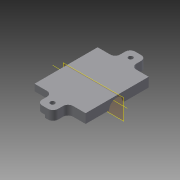
# Autodesk Inventor part: bnc-mount
Saved by Autodesk Inventor 2015 SP1 (Build 190203100, 203)
## iProperties
Created: 2015-04-03
Part Number: bnc-mount
Material: Generic
Document SubType Name: Modeling
Designer: kam42
Density: 1 g/cm^3
Appearance: Default
Author: kam42
Autodesk Inventor part; units mm, degrees
ref_plane "YZ Plane" through (0, 0, 0) normal (1, 0, 0) x (0, 1, 0)
ref_plane "XZ Plane" through (0, 0, 0) normal (0, 1, 0) x (-1, 0, 0)
ref_plane "XY Plane" through (0, 0, 0) normal (0, 0, 1) x (1, 0, 0)
sketch "Sketch1" plane through (0, 0, 0) normal (0, 0, 1) x (1, 0, 0)
  line L0 (0, 0) -> (0, 59.9999)
  line L1 (0, 59.9999) -> (45.0012, 59.9999)
  line L2 (45.0012, 59.9999) -> (45.0012, 0)
  line L3 (45.0012, 0) -> (0, 0)
  circle A0 centre (29.9999, 52.4993) radius 3.175
  circle A1 centre (29.9999, 7.5006) radius 3.175
  circle A2 centre (5.4991, 54.5008) radius 0.5842
  circle A3 centre (2.1996, 57.8002) radius 1.0541
  circle A4 centre (8.8011, 57.8002) radius 1.0541
  circle A5 centre (8.8011, 51.1988) radius 1.0541
  circle A6 centre (2.1996, 51.1988) radius 1.0541
  circle A7 centre (5.4991, 29.9999) radius 0.5842
  circle A8 centre (2.1996, 33.2994) radius 1.0541
  circle A9 centre (8.8011, 33.2994) radius 1.0541
  circle A10 centre (2.1996, 26.7005) radius 1.0541
  circle A11 centre (5.4991, 5.4991) radius 0.5842
  circle A12 centre (2.1996, 8.8011) radius 1.0541
  circle A13 centre (8.8011, 8.8011) radius 1.0541
  circle A14 centre (8.8011, 2.1996) radius 1.0541
  circle A15 centre (2.1996, 2.1996) radius 1.0541
  circle A16 centre (41.0312, 34.4602) radius 0.4496
  circle A17 centre (41.0312, 31.9202) radius 0.4496
  circle A18 centre (41.0312, 29.3802) radius 0.4496
  circle A19 centre (41.0312, 26.8402) radius 0.4496
  circle A20 centre (41.0312, 24.3002) radius 0.4496
  circle A21 centre (30.0939, 24.9352) radius 0.4496
  circle A22 centre (32.6339, 24.9352) radius 0.4496
  circle A23 centre (8.8011, 26.7005) radius 1.0541
  line L4 (45.5012, 60.4999) -> (45.5012, -0.5)
  line L5 (45.5012, -0.5) -> (-0.5, -0.5)
  line L6 (-0.5, -0.5) -> (-0.5, 60.4999)
  line L7 (-0.5, 60.4999) -> (45.5012, 60.4999)
  dimension "d0" = 0.5
  constraints: 24 centre point, 16 end point, 2 horizontal, 2 vertical, 1 coincident, 56 other
  measures "d0" distance between parallel lines of L7 L1
extrude "Extrusion1" add sketch "Sketch1" against normal blind 1 contours L0 L1 L2 L3 | A0 | A1 | A2 | A3 | A4 | A5 | A6 | A7 | A8 | A9 | A10 | A11 | A12 | A13 | A14 | A15 | A16 | A17 | A18 | A19 | A20 | A21 | A22 | A23 | L4 L5 L6 L7
sketch "Sketch2" plane through (0, 0, 0) normal (0, 0, 1) x (1, 0, 0)
  circle A0 centre (29.9999, 52.4993) radius 3.175 projected
  circle A1 centre (29.9999, 7.5006) radius 3.175 projected
  circle A2 centre (29.9999, 52.4993) radius 2.675
  circle A3 centre (29.9999, 7.5006) radius 2.675
  point P0 (0, 0)
  dimension "d6" = 0.5
  dimension "d8" = 0.5
  constraints: 2 centre point
  measures "d6" radial gap between concentric circles of A0 A2
  measures "d8" radial gap between concentric circles of A1 A3
extrude "Extrusion2" add sketch "Sketch2" along normal blind 8.25 contours A2 | A3
sketch "Sketch3" plane through (0, 0, 0) normal (0, 0, 1) x (1, 0, 0)
  line L0 (45.5012, 60.4999) -> (45.5012, -0.5) projected
  line L1 (-0.5, 60.4999) -> (45.5012, 60.4999) projected
  line L2 (-0.5, -0.5) -> (-0.5, 60.4999) projected
  line L3 (45.5012, -0.5) -> (-0.5, -0.5) projected
  line L4 (46.5012, 61.4999) -> (46.5012, -1.5)
  line L5 (46.5012, -1.5) -> (-1.5, -1.5)
  line L6 (-1.5, -1.5) -> (-1.5, 61.4999)
  line L7 (-1.5, 61.4999) -> (46.5012, 61.4999)
  line L8 (-1.5, 61.4999) -> (-4.5, 61.4999)
  line L9 (-4.5, 61.4999) -> (-4.5, -1.5)
  line L10 (-4.5, -1.5) -> (-1.5, -1.5)
  line L11 (-1.5, -1.5) -> (-1.5, 61.4999)
  point P0 (0, 0)
  dimension "d11" = 1
  dimension "d40" = 3
  constraints: 16 end point, 2 parallel, 1 horizontal, 1 perpendicular, 3 other
  measures "d11" distance between parallel lines of L1 L7
  measures "d40" distance of L9.end L10.end
extrude "Extrusion3" add sketch "Sketch3" along normal blind 16.5 and the other way blind 1
sketch "Sketch5" plane through (-4.5, -1.5, 16.5) normal (-1, 0, 0) x (0, 0, 1)
  line L0 (-16.5, 56.6743) -> (-16.5, 51.3243)
  line L1 (-16.5, 11.6756) -> (-16.5, 6.3256)
  line L2 (-16.5, 61.9999) -> (-16.5, 1)
  line L3 (-16.5, 1) -> (-16.5, 61.9999)
  circle A0 centre (-5.5, 56.0008) radius 5
  circle A1 centre (-5.5, 31.4999) radius 5
  circle A2 centre (-5.5, 6.9991) radius 5
  line L4 (-10.5, 56.0008) -> (-10.5, 6.9991) construction
  point P0 (-16.5, 1.5)
  point P1 (-16.5, 31.4999)
  point P2 (-16.5, 56.0008)
  point P3 (-16.5, 6.9991)
  point P4 (-16.5, 31.4999)
  dimension "d16" = 10
  dimension "d18" = 10
  dimension "d17" = 10
  dimension "d20" = 6
  constraints: 10 end point, 5 horizontal alignment, 2 vertical, 2 vertical alignment, 1 centre point, 1 midpoint, 4 other
  measures "d17" diameter of A1
  measures "d20" distance between parallel lines of L2 L4
sketch "Sketch6" plane through (0, 0, 0) normal (0, 0, 1) x (1, 0, 0)
  line L0 (-0.5, -0.5) -> (-0.5, 60.4999) projected
  line L1 (-0.5, 48.2508) -> (11.5, 48.2508)
  line L2 (11.5, 48.2508) -> (11.5, 36.2508)
  line L3 (11.5, 36.2508) -> (-0.5, 36.2508)
  line L4 (-0.5, 36.2508) -> (-0.5, 48.2508)
  line L5 (-0.5, 23.7499) -> (11.5, 23.7499)
  line L6 (11.5, 23.7499) -> (11.5, 11.7499)
  line L7 (11.5, 11.7499) -> (-0.5, 11.7499)
  line L8 (-0.5, 11.7499) -> (-0.5, 23.7499)
  line L9 (-0.5, 48.2508) -> (11.5, 36.2508) construction
  line L10 (-0.5, 36.2508) -> (11.5, 48.2508) construction
  line L11 (-0.5, 23.7499) -> (11.5, 11.7499) construction
  line L12 (11.5, 23.7499) -> (-0.5, 11.7499) construction
  point P0 (0, 0)
  point P1 (5.5, 42.2508)
  point P2 (5.5, 17.7499)
  point P3 (5.4991, 29.9999)
  point P4 (5.4991, 54.5008)
  dimension "d21" = 12
  dimension "d22" = 12
  dimension "d23" = 12
  dimension "d24" = 12.25
  dimension "d25" = 12.25
  constraints: 24 end point, 4 parallel, 4 point on line, 3 perpendicular, 2 horizontal, 2 midpoint
  measures "d21" distance of L5.end L6.end
  measures "d22" distance of L1.end L2.end
  measures "d23" distance of L5.start L5.end
  measures "d24" distance of point (5.499, 30) point (5.5, 17.75)
  measures "d25" distance of point (5.499, 54.501) point (5.5, 42.251)
extrude "Extrusion4" add sketch "Sketch6" along normal blind 3.75
extrude "Extrusion5" cut sketch "Sketch5" against normal up to surface (4 mm away)
sketch "Sketch7" plane through (46.5012, -1.5, 16.5) normal (1, 0, 0) x (0, 0, -1)
  line L0 (16.5, 61.9999) -> (16.5, 1) projected
  circle A0 centre (8.5, 30.8802) radius 2
  point P0 (16.5, 1.5)
  point P1 (16.5, 30.8802)
  point P2 (10.5, 30.8802)
  dimension "d33" = 4
  dimension "d32" = 6
  constraints: 1 horizontal alignment, 2 other
  measures "d32" distance of point (10.5, 30.88) point (16.5, 30.88)
extrude "Extrusion6" cut sketch "Sketch7" against normal up to surface (1 mm away)
sketch "Sketch8" plane through (0, 0, 16.5) normal (0, 0, 1) x (1, 0, 0)
  line L0 (45.5012, -0.5) -> (-0.5, -0.5) projected
  line L1 (-0.5, -0.5) -> (-0.5, 60.4999) projected
  line L2 (-0.5, 60.4999) -> (45.5012, 60.4999) projected
  line L3 (45.5012, 60.4999) -> (45.5012, -0.5) projected
  line L4 (46.5012, 61.4999) -> (-4.5, 61.4999) projected
  line L5 (-4.5, 61.4999) -> (-4.5, -1.5) projected
  line L6 (-4.5, -1.5) -> (46.5012, -1.5) projected
  line L7 (46.5012, -1.5) -> (46.5012, 61.4999) projected
  point P0 (0, 0)
extrude "Extrusion8" add sketch "Sketch8" along normal blind 1 contours L0 L1 L2 L3 | L7 L6 L5 L4
ref_plane "Work Plane1" through (-3.5, -1.5, 16.5) normal (0, -1, 0) x (1, 0, 0)
sketch "Sketch10" plane through (-3.5, -1.5, 16.5) normal (0, -1, 0) x (1, 0, 0)
  line L0 (24.5006, -5.5) -> (24.5006, -8.25)
  line L1 (50.0012, -8.25) -> (24.5006, -8.25)
  line L2 (-1, -5.5) -> (24.5006, -5.5)
  line L3 (50.0012, -6.5) -> (50.0012, -10.5) projected
  line L4 (-1, -10.5) -> (-1, -0.5) projected
  line L5 (3, -0.5) -> (3, -10.5) projected
  constraints: 6 end point, 1 horizontal, 1 parallel
split body "Split1" sketch "Sketch10" result two bodies curves L1 L0 L2 first body at (12.5004, 40.4999, -0.5)
ref_plane "Work Plane2" through (46.5012, -0.5, 0) normal (1, 0, 0) x (0, 0, -1)
sketch "Sketch13" plane through (46.5012, -0.5, 0) normal (1, 0, 0) x (0, 0, -1)
  line L0 (-8.25, -1) -> (-8.25, 27.8959) projected
  line L1 (-8.25, -1) -> (1, -1) projected
  line L2 (1, 61.9999) -> (1, -1) projected
  line L3 (1, 61.9999) -> (-8.25, 61.9999) projected
  line L4 (-8.25, 31.8645) -> (-8.25, 61.9999) projected
  arc A0 (-6, 29.8802) -> (-8.25, 31.8645) centre (-8, 29.8802) ccw projected
  arc A1 (-8.25, 27.8959) -> (-6, 29.8802) centre (-8, 29.8802) ccw projected
  circle A2 centre (-8, 29.8802) radius 5
  circle A3 centre (-8, 29.8802) radius 2
  line L5 (-8.25, 27.8959) -> (-8.25, 0) projected
  line L6 (-8.25, 24.8864) -> (-8.25, 27.8959)
  line L7 (-8.25, 31.8645) -> (-8.25, 34.8739)
  line L8 (-8.25, 31.8645) -> (-8.25, 61.9999) projected
  dimension "d63" = 10
  constraints: 4 end point, 2 centre point, 2 coincident, 2 point on circle, 2 point on line, 1 collinear
  measures "d63" diameter of A2
extrude "Extrusion14" add sketch "Sketch13" along normal blind 4 contours L0 A1 A0 L4 A2 bodies 2
sketch "Sketch18" plane through (46.5012, -1.5, 17.5) normal (1, 0, 0) x (0, 0, -1)
  line L0 (9.25, 0) -> (9.25, 28.8959) projected
  arc A0 (9.25, 32.8645) -> (9.25, 28.8959) centre (9.5, 30.8802) ccw projected
  line L1 (9.25, 32.8645) -> (9.25, 62.9999) projected
  arc A1 (9.25, 25.8864) -> (9.25, 35.8739) centre (9.5, 30.8802) ccw projected
  circle A2 centre (9.5, 30.8802) radius 7.5
  circle A3 centre (9.5, 30.8802) radius 2
  line L2 (9.25, 25.8864) -> (9.25, 28.8959)
  line L3 (9.25, 28.8959) -> (9.25, 1) projected
  line L4 (9.25, 35.8739) -> (9.25, 32.8645)
  point P0 (17.5, 1.5)
  dimension "d140" = 15
  constraints: 4 end point, 2 centre point, 2 coincident, 2 collinear
  measures "d140" diameter of A2
sketch "Sketch21" plane through (-4.5, -1.5, -1) normal (0, -1, 0) x (1, 0, 0)
  line L0 (25.5006, 9.25) -> (51.0012, 9.25) projected
  line L1 (25.5006, 12) -> (25.5006, 9.25) projected
  line L2 (51.0012, 0) -> (0, 0) projected
  line L3 (4, 12) -> (25.5006, 12) projected
  line L4 (17.5006, 12) -> (25.5006, 12)
  line L5 (33.5006, 9.25) -> (33.5006, 0)
  line L6 (33.5006, 0) -> (17.5006, 0)
  line L7 (17.5006, 0) -> (17.5006, 12)
  point P0 (4.5, 1)
  dimension "d78" = 8
  dimension "d79" = 8
  constraints: 8 end point, 4 point on line, 2 parallel, 1 horizontal, 1 perpendicular
  measures "d78" distance between parallel lines of L1 L7
  measures "d79" distance between parallel lines of L5 L1
extrude "Extrusion18" add sketch "Sketch21" along normal blind 15 bodies 2
sketch "Sketch22" plane through (-4.5, -1.5, 17.5) normal (0, -1, 0) x (1, 0, 0)
  line L0 (25.5006, -6.5) -> (25.5006, -9.25) projected
  line L1 (25.5006, -9.25) -> (25.5006, -6.5) projected
  line L2 (25.5006, -6.5) -> (17.5006, -6.5) projected
  line L3 (17.5006, -6.5) -> (17.5006, -18.5) projected
  line L4 (17.5006, -18.5) -> (33.5006, -18.5) projected
  line L5 (33.5006, -18.5) -> (33.5006, -9.25) projected
  line L6 (33.5006, -9.25) -> (25.5006, -9.25) projected
  line L7 (51.0012, 0) -> (0, 0) projected
  line L8 (33.5006, -9.25) -> (25.5006, -9.25)
  line L9 (17.5006, -6.5) -> (17.5006, 0)
  line L10 (17.5006, 0) -> (33.5006, 0)
  line L11 (33.5006, 0) -> (33.5006, -9.25)
  line L12 (17.5006, -6.5) -> (25.5006, -6.5)
  point P0 (4.5, -17.5)
  constraints: 10 end point, 3 point on line, 2 horizontal, 2 parallel, 1 perpendicular
extrude "Extrusion19" add sketch "Sketch22" along normal blind 15 contours L2 L9 L7 L11 L6 L0 bodies 3
sketch "Sketch23" plane through (0, 0, 17.5) normal (0, 0, 1) x (1, 0, 0)
  line L0 (21.0006, -0.5) -> (21.0006, -16.5) projected
  point P0 (0, 0)
  point P1 (21.0006, -9)
  constraints: 1 point on line
hole "Hole1" at (21.0006, -9, 17.5) direction (0, 0, -1) diameter 4.4958 end through all bodies 3 2
sketch "Sketch24" plane through (0, 0, -1) normal (0, 0, -1) x (-1, 0, 0)
  circle A0 centre (-21.0006, -9) radius 2.2479 projected
  line L0 (-25.3381, -11.5367) -> (-25.3662, -6.5119)
  line L1 (-25.3662, -6.5119) -> (-21.0287, -3.9752)
  line L2 (-21.0287, -3.9752) -> (-16.663, -6.4633)
  line L3 (-16.663, -6.4633) -> (-16.635, -11.4881)
  line L4 (-16.635, -11.4881) -> (-20.9725, -14.0248)
  line L5 (-20.9725, -14.0248) -> (-25.3381, -11.5367)
  point P0 (0, 0)
  dimension "d91" = 8.7312
  constraints: 12 end point, 1 coincident, 13 other
  measures "d91" horizontal distance of L0.end L3.end
extrude "Extrusion20" cut sketch "Sketch24" against normal blind 3.175 bodies 2
ref_plane "Work Plane4" through (-4.5, 29.9999, 11) normal (0, -1, 0) x (1, 0, 0)
mirror "Mirror2" about plane through (-4.5, 29.9999, 11) normal (0, -1, 0) of "Extrusion18", "Hole1", "Extrusion20" bodies 2
mirror "Mirror3" about plane through (-4.5, 29.9999, 11) normal (0, -1, 0) of "Extrusion19", "Hole1" bodies 3
fillet "Fillet4" radius 5 16 edges at (13.0006, -1.5, 5) (13.0006, -16.5, 5) (29.0006, -16.5, 3.625) (29.0006, -1.5, 3.625) (13.0006, 61.4999, 5) (13.0006, 76.4999, 5) (29.0006, 76.4999, 3.625) (29.0006, 61.4999, 3.625) (13.0006, -1.5, 14.25) (13.0006, -16.5, 14.25) (29.0006, -16.5, 12.875) (29.0006, -1.5, 12.875) (13.0006, 61.4999, 14.25) (13.0006, 76.4999, 14.25) (29.0006, 76.4999, 12.875) (29.0006, 61.4999, 12.875)
sketch "Sketch25" plane through (0, 0, 0) normal (0, 0, 1) x (1, 0, 0)
  circle A0 centre (29.9999, 7.5006) radius 2.675 projected
  circle A1 centre (29.9999, 52.4993) radius 2.675 projected
  circle A2 centre (29.9999, 52.4993) radius 5
  circle A3 centre (29.9999, 7.5006) radius 5
  point P0 (0, 0)
  dimension "d96" = 10
  dimension "d97" = 10
  constraints: 2 centre point, 2 coincident
  measures "d96" diameter of A2
  measures "d97" diameter of A3
extrude "Extrusion21" add sketch "Sketch25" along normal blind 3.75 bodies 2
sketch "Sketch26" plane through (29.9999, 7.5006, 8.25) normal (0, 0, 1) x (1, 0, 0)
  circle A0 centre (0, 0) radius 2.675 projected
  circle A1 centre (0, 44.9986) radius 2.675 projected
  point P0 (-29.9999, -7.5006)
  constraints: 2 coincident
hole "Hole2" at (29.9999, 7.5006, 8.25) at (29.9999, 52.4993, 8.25) direction (0, 0, -1) diameter 3 depth 6 tip angle 118 bodies 2
sketch "Sketch29" plane through (0, 0, -1) normal (0, 0, -1) x (-1, 0, 0)
  arc A0 (-24.0006, 76.4999) -> (-29.0006, 71.4999) centre (-24.0006, 71.4999) ccw projected
  line L0 (-29.0006, 66.4999) -> (-29.0006, 71.4999) projected
  arc A1 (-34.0006, 61.4999) -> (-29.0006, 66.4999) centre (-34.0006, 66.4999) ccw projected
  line L1 (-34.0006, 61.4999) -> (-46.5012, 61.4999) projected
  line L2 (-46.5012, 61.4999) -> (-46.5012, -1.5) projected
  line L3 (-46.5012, -1.5) -> (-34.0006, -1.5) projected
  arc A2 (-29.0006, -6.5) -> (-34.0006, -1.5) centre (-34.0006, -6.5) ccw projected
  line L4 (-29.0006, -6.5) -> (-29.0006, -11.5) projected
  arc A3 (-29.0006, -11.5) -> (-24.0006, -16.5) centre (-24.0006, -11.5) ccw projected
  line L5 (-18.0006, -16.5) -> (-24.0006, -16.5) projected
  arc A4 (-18.0006, -16.5) -> (-13.0006, -11.5) centre (-18.0006, -11.5) ccw projected
  line L6 (-13.0006, -6.5) -> (-13.0006, -11.5) projected
  arc A5 (-8.0006, -1.5) -> (-13.0006, -6.5) centre (-8.0006, -6.5) ccw projected
  line L7 (-8.0006, -1.5) -> (4.5, -1.5) projected
  line L8 (4.5, -1.5) -> (4.5, 61.4999) projected
  line L9 (4.5, 61.4999) -> (-8.0006, 61.4999) projected
  arc A6 (-13.0006, 66.4999) -> (-8.0006, 61.4999) centre (-8.0006, 66.4999) ccw projected
  line L10 (-13.0006, 66.4999) -> (-13.0006, 71.4999) projected
  arc A7 (-13.0006, 71.4999) -> (-18.0006, 76.4999) centre (-18.0006, 71.4999) ccw projected
  line L11 (-18.0006, 76.4999) -> (-24.0006, 76.4999) projected
  line L12 (7, 63.9999) -> (7, -4)
  line L13 (7, -4) -> (-8.0006, -4)
  arc A8 (-8.0006, -4) -> (-10.5006, -6.5) centre (-8.0006, -6.5) ccw
  line L14 (-10.5006, -6.5) -> (-10.5006, -11.5)
  arc A9 (-18.0006, -19) -> (-10.5006, -11.5) centre (-18.0006, -11.5) ccw
  line L15 (-18.0006, -19) -> (-24.0006, -19)
  arc A10 (-31.5006, -11.5) -> (-24.0006, -19) centre (-24.0006, -11.5) ccw
  line L16 (-31.5006, -11.5) -> (-31.5006, -6.5)
  arc A11 (-31.5006, -6.5) -> (-34.0006, -4) centre (-34.0006, -6.5) ccw
  line L17 (-34.0006, -4) -> (-49.0012, -4)
  line L18 (-49.0012, -4) -> (-49.0012, 63.9999)
  line L19 (-49.0012, 63.9999) -> (-34.0006, 63.9999)
  arc A12 (-34.0006, 63.9999) -> (-31.5006, 66.4999) centre (-34.0006, 66.4999) ccw
  line L20 (-31.5006, 66.4999) -> (-31.5006, 71.4999)
  arc A13 (-24.0006, 78.9999) -> (-31.5006, 71.4999) centre (-24.0006, 71.4999) ccw
  line L21 (-24.0006, 78.9999) -> (-18.0006, 78.9999)
  arc A14 (-10.5006, 71.4999) -> (-18.0006, 78.9999) centre (-18.0006, 71.4999) ccw
  line L22 (-10.5006, 71.4999) -> (-10.5006, 66.4999)
  arc A15 (-10.5006, 66.4999) -> (-8.0006, 63.9999) centre (-8.0006, 66.4999) ccw
  line L23 (-8.0006, 63.9999) -> (7, 63.9999)
  point P0 (0, 0)
  dimension "d109" = 2.5
  constraints: 24 end point, 16 point on circle, 8 centre point, 19 other
  measures "d109" distance between parallel lines of L12 L8
extrude "Extrusion22" add sketch "Sketch29" against normal blind 18.5 bodies 2
sketch "Sketch31" plane through (49.0012, -4, -1) normal (1, 0, 0) x (0, 0, -1)
  arc A0 (-9.25, 28.3864) -> (-9.25, 38.3739) centre (-9, 33.3802) ccw projected
  arc A1 (-9.25, 31.3959) -> (-9.25, 35.3645) centre (-9, 33.3802) ccw projected
  circle A2 centre (-9, 33.3802) radius 2
  circle A3 centre (-9, 33.3802) radius 6
  line L0 (-9.25, 28.3864) -> (-9.25, 27.3854)
  line L1 (-9.25, 31.3959) -> (-9.25, 3.5) projected
  line L2 (-9.25, 38.3739) -> (-9.25, 39.375)
  line L3 (-9.25, 64.4999) -> (-9.25, 35.3645) projected
  point P0 (-1, 4)
  dimension "d117" = 1
  constraints: 4 end point, 2 centre point, 2 coincident, 2 point on circle, 2 point on line, 1 concentric
  measures "d117" radial gap between concentric circles of A0 A3
extrude "Extrusion24" cut sketch "Sketch31" against normal blind 18.5 contours L0 A3 L2 L3 A2 L1 | A2 A1 bodies 2
sketch "Sketch33" plane through (-7, -4, -1) normal (-1, 0, 0) x (0, 0, 1)
  line L0 (12, 14.4991) -> (12, 28.9999) projected
  arc A0 (12, 14.4991) -> (12, 4.4991) centre (12, 9.4991) ccw projected
  line L1 (12, 3.5) -> (12, 4.4991) projected
  line L2 (1, 3.5) -> (12, 3.5) projected
  line L3 (1, 3.5) -> (1, 15.7499) projected
  line L4 (1, 15.7499) -> (4.75, 15.7499) projected
  line L5 (4.75, 15.7499) -> (4.75, 27.7499) projected
  line L6 (4.75, 27.7499) -> (1, 27.7499) projected
  line L7 (1, 27.7499) -> (1, 40.2508) projected
  line L8 (1, 40.2508) -> (4.75, 40.2508) projected
  line L9 (4.75, 40.2508) -> (4.75, 52.2508) projected
  line L10 (4.75, 52.2508) -> (1, 52.2508) projected
  line L11 (1, 52.2508) -> (1, 64.4999) projected
  line L12 (1, 64.4999) -> (12, 64.4999) projected
  line L13 (12, 63.5008) -> (12, 64.4999) projected
  arc A1 (12, 63.5008) -> (12, 53.5008) centre (12, 58.5008) ccw projected
  line L14 (12, 38.9999) -> (12, 53.5008) projected
  arc A2 (12, 38.9999) -> (12, 28.9999) centre (12, 33.9999) ccw projected
  circle A3 centre (12, 58.5008) radius 5.4
  circle A4 centre (12, 33.9999) radius 5.4
  circle A5 centre (12, 9.4991) radius 5.4
  line L15 (12, 63.5008) -> (12, 64.0003)
  line L16 (12, 63.5008) -> (12, 64.4999) projected
  line L17 (12, 53.5008) -> (12, 53.1008)
  line L18 (12, 38.9999) -> (12, 53.5008) projected
  line L19 (12, 39.3999) -> (12, 38.9999)
  line L20 (12, 28.9999) -> (12, 28.5999)
  line L21 (12, 14.4991) -> (12, 28.9999) projected
  line L22 (12, 14.8991) -> (12, 14.4991)
  line L23 (12, 4.4991) -> (12, 4.0991)
  arc A6 (12, 63.5008) -> (12, 53.5008) centre (12, 58.5008) ccw
  arc A7 (12, 38.9999) -> (12, 28.9999) centre (12, 33.9999) ccw
  arc A8 (12, 14.4991) -> (12, 4.4991) centre (12, 9.4991) ccw
  point P0 (1, 4)
  dimension "d118" = 0.4
  dimension "d119" = 0.4
  dimension "d120" = 0.4
  constraints: 15 end point, 10 point on circle, 6 coincident, 5 centre point, 5 point on line, 2 collinear, 2 midpoint, 1 concentric, 1 vertical alignment, 2 other
  measures "d118" radial gap between concentric circles of A0 A5
  measures "d119" radial gap between concentric circles of A4 A2
extrude "Extrusion25" cut sketch "Sketch33" against normal blind 18.5 contours A0 L1 A5 L0 | L0 A5 L1 A0 | A4 L14 A2 L0 | L0 A2 L14 A4 | A3 L13 A1 L14 | L14 A1 L13 A3 bodies 2
extrude "Extrusion26" cut sketch "Sketch18" against normal up to surface (1 mm away) contours L0 A2 L1 A0 | A1 L1 A2 L0 bodies 3
sketch "Sketch35" plane through (0, 0, 16.5) normal (0, 0, -1) x (-1, 0, 0)
  line L0 (0.5, 60.4999) -> (-45.5012, 60.4999) projected
  line L1 (-45.5012, 60.4999) -> (-45.5012, -0.5) projected
  line L2 (-45.5012, -0.5) -> (0.5, -0.5) projected
  line L3 (-45.5012, 21.8843) -> (-46.5012, 21.8843) projected
  line L4 (-46.5012, -1.5) -> (-46.5012, 21.8843) projected
  line L5 (-34.0006, -1.5) -> (-46.5012, -1.5) projected
  arc A0 (-29.0006, -6.5) -> (-34.0006, -1.5) centre (-34.0006, -6.5) ccw projected
  line L6 (-29.0006, -6.5) -> (-29.0006, -11.5) projected
  arc A1 (-29.0006, -11.5) -> (-24.0006, -16.5) centre (-24.0006, -11.5) ccw projected
  line L7 (-21.0006, -16.5) -> (-24.0006, -16.5) projected
  line L8 (-21.0006, -11.2479) -> (-21.0006, -16.5) projected
  arc A2 (-21.0006, -6.7521) -> (-21.0006, -11.2479) centre (-21.0006, -9) ccw projected
  line L9 (-21.0006, -0.5) -> (-21.0006, -6.7521) projected
  line L10 (-45.5012, -0.5) -> (-21.0006, -0.5) projected
  line L11 (-45.5012, 21.8843) -> (-45.5012, -0.5) projected
  line L12 (-46.5012, 36.876) -> (-45.5012, 36.876) projected
  line L13 (-45.5012, 60.4999) -> (-45.5012, 36.876) projected
  line L14 (-21.0006, 60.4999) -> (-45.5012, 60.4999) projected
  line L15 (-21.0006, 60.4999) -> (-21.0006, 66.752) projected
  arc A3 (-21.0006, 71.2478) -> (-21.0006, 66.752) centre (-21.0006, 68.9999) ccw projected
  line L16 (-21.0006, 71.2478) -> (-21.0006, 76.4999) projected
  line L17 (-21.0006, 76.4999) -> (-24.0006, 76.4999) projected
  arc A4 (-24.0006, 76.4999) -> (-29.0006, 71.4999) centre (-24.0006, 71.4999) ccw projected
  line L18 (-29.0006, 66.4999) -> (-29.0006, 71.4999) projected
  arc A5 (-34.0006, 61.4999) -> (-29.0006, 66.4999) centre (-34.0006, 66.4999) ccw projected
  line L19 (-46.5012, 61.4999) -> (-34.0006, 61.4999) projected
  line L20 (-46.5012, 36.876) -> (-46.5012, 61.4999) projected
  line L21 (-21.0006, -0.5) -> (-45.5012, -0.5)
  line L22 (-45.5012, -0.5) -> (-45.5012, 0.5)
  line L23 (-44.5012, 0.5) -> (-21.0006, 0.5)
  line L24 (-21.0006, 0.5) -> (-21.0006, -0.5)
  line L25 (-21.0006, 60.4999) -> (-45.5012, 60.4999) projected
  line L26 (-44.5012, 0.5) -> (-44.5012, 59.4999)
  line L27 (-44.5012, 60.4999) -> (-45.5012, 60.4999)
  line L28 (-45.5012, 60.4999) -> (-45.5012, 0.5)
  line L29 (-44.5012, 60.4999) -> (-21.0006, 60.4999)
  line L30 (-21.0006, 60.4999) -> (-21.0006, 59.4999)
  line L31 (-21.0006, 59.4999) -> (-44.5012, 59.4999)
  point P0 (0, 0)
  dimension "d126" = 1
  dimension "d127" = 1
  dimension "d128" = 1
  constraints: 20 end point, 4 parallel, 3 point on line, 2 horizontal, 2 perpendicular
  measures "d126" distance between parallel lines of L1 L26
  measures "d127" distance between parallel lines of L2 L23
  measures "d128" distance between parallel lines of L0 L31
extrude "Extrusion27" add sketch "Sketch35" along normal up to surface (8.25 mm away) contours L30 L31 L26 L23 L24 L2 L1 L0 bodies 3
sketch "Sketch36" plane through (0, 0, 16.5) normal (0, 0, -1) x (-1, 0, 0)
  arc A0 (-18.0006, -16.5) -> (-13.0006, -11.5) centre (-18.0006, -11.5) ccw projected
  line L0 (-13.0006, -6.5) -> (-13.0006, -11.5) projected
  arc A1 (-8.0006, -1.5) -> (-13.0006, -6.5) centre (-8.0006, -6.5) ccw projected
  line L1 (4.5, -1.5) -> (-8.0006, -1.5) projected
  line L2 (4.5, 0.4991) -> (4.5, -1.5) projected
  line L3 (0.5, 0.4991) -> (4.5, 0.4991) projected
  line L4 (0.5, -0.5) -> (0.5, 0.4991) projected
  line L5 (-21.0006, -0.5) -> (0.5, -0.5) projected
  line L6 (-21.0006, -0.5) -> (-21.0006, -6.7521) projected
  arc A2 (-21.0006, -11.2479) -> (-21.0006, -6.7521) centre (-21.0006, -9) ccw projected
  line L7 (-21.0006, -11.2479) -> (-21.0006, -16.5) projected
  line L8 (-18.0006, -16.5) -> (-21.0006, -16.5) projected
  arc A3 (-13.0006, 71.4999) -> (-18.0006, 76.4999) centre (-18.0006, 71.4999) ccw projected
  line L9 (-18.0006, 76.4999) -> (-21.0006, 76.4999) projected
  line L10 (-21.0006, 71.2478) -> (-21.0006, 76.4999) projected
  arc A4 (-21.0006, 66.752) -> (-21.0006, 71.2478) centre (-21.0006, 68.9999) ccw projected
  line L11 (-21.0006, 60.4999) -> (-21.0006, 66.752) projected
  line L12 (0.5, 60.4999) -> (-21.0006, 60.4999) projected
  line L13 (0.5, 59.5008) -> (0.5, 60.4999) projected
  line L14 (4.5, 59.5008) -> (0.5, 59.5008) projected
  line L15 (4.5, 61.4999) -> (4.5, 59.5008) projected
  line L16 (-8.0006, 61.4999) -> (4.5, 61.4999) projected
  arc A5 (-13.0006, 66.4999) -> (-8.0006, 61.4999) centre (-8.0006, 66.4999) ccw projected
  line L17 (-13.0006, 66.4999) -> (-13.0006, 71.4999) projected
  line L18 (0.5, 0.4991) -> (-21.0006, 0.4991)
  line L19 (-21.0006, 0.4991) -> (-21.0006, -0.5)
  line L20 (-21.0006, -0.5) -> (0.5, -0.5)
  line L21 (0.5, -0.5) -> (0.5, 0.4991)
  line L22 (0.5, 59.5008) -> (-21.0006, 59.5008)
  line L23 (-21.0006, 59.5008) -> (-21.0006, 60.4999)
  line L24 (-21.0006, 60.4999) -> (0.5, 60.4999)
  line L25 (0.5, 60.4999) -> (0.5, 59.5008)
  point P0 (0, 0)
  constraints: 16 end point, 4 parallel, 2 horizontal, 2 perpendicular
extrude "Extrusion28" add sketch "Sketch36" along normal up to surface (5.5 mm away) contours L19 L18 L4 L5 | L12 L13 L22 L23 bodies 3
sketch "Sketch37" plane through (45.5012, 29.3802, 8) normal (1, 0, 0) x (0, 0, -1)
  arc A0 (-0.25, 7.4958) -> (-0.25, -7.4958) centre (0, 0) ccw projected
  line L0 (-0.25, -7.4958) -> (-0.25, 7.4958) projected
  point P0 (8, -29.3802)
extrude "Extrusion29" cut sketch "Sketch37" against normal up to surface (1 mm away) bodies 3
sketch "Sketch38" plane through (50.5012, -0.5, 0) normal (1, 0, 0) x (0, 0, -1)
  line L0 (-8.25, 27.8959) -> (-8.25, 24.8864) projected
  arc A0 (-8.25, 24.8864) -> (-8.25, 34.8739) centre (-8, 29.8802) ccw projected
  line L1 (-8.25, 34.8739) -> (-8.25, 31.8645) projected
  arc A1 (-8.25, 27.8959) -> (-8.25, 31.8645) centre (-8, 29.8802) ccw projected
  arc A2 (-8.25, 20.8623) -> (-8.25, 38.898) centre (-8, 29.8802) ccw
  line L2 (-8.25, 24.8864) -> (-8.25, 20.8623)
  line L3 (-8.25, -1) -> (-8.25, 23.8854) projected
  line L4 (-8.25, 34.8739) -> (-8.25, 38.898)
  line L5 (-8.25, 35.875) -> (-8.25, 61.9999) projected
  point P0 (0, 0.5)
  constraints: 4 end point, 2 point on circle, 2 point on line, 1 centre point, 1 coincident
extrude "Extrusion30" add sketch "Sketch38" against normal blind 3 and the other way blind 10 bodies 2
fillet "Fillet5" radius 2 5 edges at (49.0012, 36.0594, 1.936) (49.0012, 22.701, 1.936) (49.0012, 21.8739, 8.25) (49.0012, 36.8865, 8.25) (60.5012, 29.3802, -1.0213)
body "Solid2"
body "Solid3"
